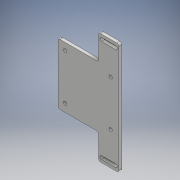
# Autodesk Inventor part: RTK Mount
Saved by Autodesk Inventor 2018 (Build 220112000, 112)
## iProperties
Created: 2017-06-29
Part Number: RTK Mount
Material: Generic
Document SubType Name: Modeling
Designer: klyu
Density: 1 g/cm^3
Appearance: Default
Author: klyu
Autodesk Inventor part; units mm, degrees
ref_plane "YZ Plane" through (0, 0, 0) normal (1, 0, 0) x (0, 1, 0)
ref_plane "XZ Plane" through (0, 0, 0) normal (0, 1, 0) x (-1, 0, 0)
ref_plane "XY Plane" through (0, 0, 0) normal (0, 0, 1) x (1, 0, 0)
sketch "Sketch1" plane through (0, 0, 0) normal (0, 1, 0) x (-1, 0, 0)
  line L0 (0, 0) -> (20, 0)
  line L1 (20, 0) -> (20, -110)
  line L2 (20, -110) -> (0, -110)
  line L3 (0, -110) -> (0, 0)
  line L4 (17, -103.85) -> (3, -103.85)
  arc A0 (3, -103.85) -> (3, -107.15) centre (3, -105.5) ccw
  line L5 (17, -107.15) -> (3, -107.15)
  arc A1 (17, -107.15) -> (17, -103.85) centre (17, -105.5) ccw
  line L6 (17, -2.85) -> (3, -2.85)
  arc A2 (3, -2.85) -> (3, -6.15) centre (3, -4.5) ccw
  line L7 (17, -6.15) -> (3, -6.15)
  arc A3 (17, -6.15) -> (17, -2.85) centre (17, -4.5) ccw
  line L8 (20, -25) -> (60, -25)
  line L9 (60, -25) -> (60, -85)
  line L10 (60, -85) -> (20, -85)
  circle A4 centre (53, -77) radius 1.65
  circle A5 centre (53, -32) radius 1.65
  circle A6 centre (8, -32) radius 1.65
  circle A7 centre (8, -77) radius 1.65
  line L11 (53, -32) -> (8, -32)
  dimension "d0" = 110
  dimension "d1" = 20
  dimension "d3" = 3.3
  dimension "d5" = 3.3
  dimension "d8" = 2.85
  dimension "d9" = 3
  dimension "d10" = 3
  dimension "d11" = 3
  dimension "d12" = 3
  dimension "d16" = 101
  dimension "d17" = 3.3
  dimension "d18" = 60
  dimension "d19" = 60
  dimension "d20" = 25
  dimension "d21" = 3.3
  dimension "d22" = 3.3
  dimension "d23" = 3.3
  dimension "d24" = 45
  dimension "d25" = 45
  dimension "d26" = 45
  dimension "d27" = 45
  dimension "d28" = 7
  dimension "d29" = 7
  dimension "d30" = 7
  constraints: 24 end point, 10 point on circle, 8 centre point, 8 tangent, 6 horizontal, 3 perpendicular, 2 parallel, 2 point on line
  measures "d0" distance between parallel lines of L2 L0
  measures "d1" distance between parallel lines of L1 L3
  measures "d3" distance between parallel lines of L5 L4
  measures "d5" distance between parallel lines of L7 L6
  measures "d8" distance between parallel lines of L2 L5
  measures "d9" distance from line of L1 A1.centre
  measures "d10" distance from line of L3 A0.centre
  measures "d11" distance from line of L1 A3.centre
  measures "d12" distance from line of A2.centre L3
  measures "d16" distance of A1.centre A3.centre
  measures "d17" diameter of A4
  measures "d18" distance between parallel lines of L10 L8
  measures "d19" distance between parallel lines of L3 L9
  measures "d20" distance between parallel lines of L2 L10
  measures "d21" diameter of A5
  measures "d22" diameter of A6
  measures "d23" diameter of A7
  measures "d24" distance of A4.centre L11.start
  measures "d25" distance of A7.centre A4.centre
  measures "d26" distance of L11.end A7.centre
  measures "d27" distance of L11.start L11.end
  measures "d28" distance from line of L8 L11.start
  measures "d29" distance from line of L9 L11.start
  measures "d30" distance from line of L9 A4.centre
extrude "Extrusion2" add sketch "Sketch1" along normal blind 3
fillet "Fillet2" radius 2 8 edges at (0, 1.5, 0) (0, 1.5, -110) (-20, 1.5, -110) (-20, 1.5, -85) (-60, 1.5, -85) (-60, 1.5, -25) (-20, 1.5, -25) (-20, 1.5, 0)
body "Solid2"
